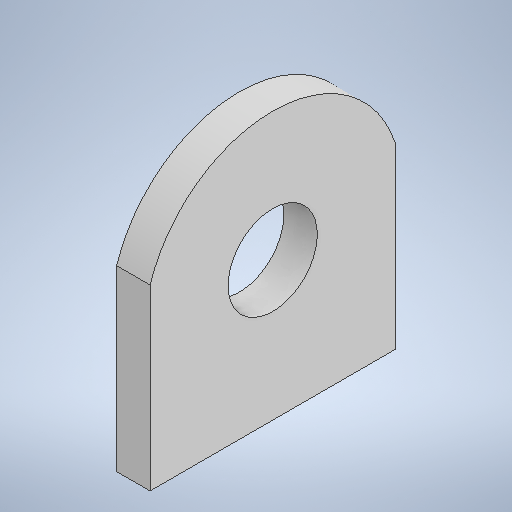
# Autodesk Inventor part: side
Saved by Autodesk Inventor 2025.2 (Build 292293000, 293)
## iProperties
Created: 2025-09-04
Part Number: side
Material: Generic
Document SubType Name: Modeling
Designer: User
Density: 1 g/cm^3
Appearance: Default
Mass: 5.16926 g
Surface Area: 29.8894 cm^2
Volume: 5.16926 cm^3
Author: User
Autodesk Inventor part; units mm, degrees
ref_plane "YZ Plane" through (0, 0, 0) normal (1, 0, 0) x (0, 1, 0)
ref_plane "XZ Plane" through (0, 0, 0) normal (0, 1, 0) x (-1, 0, 0)
ref_plane "XY Plane" through (0, 0, 0) normal (0, 0, 1) x (1, 0, 0)
sketch "Sketch1" plane through (0, 0, 0) normal (1, 0, 0) x (0, 1, 0)
  line L0 (25.3575, 17.457) -> (-0.0425, 17.457)
  line L1 (-0.0425, 17.457) -> (-0.0425, -17.468)
  line L2 (-0.0425, -17.468) -> (25.3575, -17.468)
  arc A0 (25.3575, -17.468) -> (25.3575, 17.457) centre (19.702, -0.0055) ccw
  circle A1 centre (19.702, -0.0055) radius 6.3491
  dimension "d1" = 34.925
  constraints: 6 end point, 2 centre point, 2 point on circle, 1 coincident, 1 horizontal, 1 parallel, 1 perpendicular
  measures "d1" distance between parallel lines of L0 L2
extrude "Extrusion1" add sketch "Sketch1" along normal blind 4.7625
body "Solid1"
